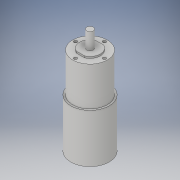
# Autodesk Inventor part: IG42-017
Saved by Autodesk Inventor 2019 (Build 230136000, 136)
## iProperties
Created: 2018-10-30
Part Number: IG42-017
Material: 一般
Document SubType Name: Modeling
Designer: kouki
Density: 1 g/cm^3
Appearance: 既定
Author: kouki
Autodesk Inventor part; units mm, degrees
ref_plane "YZ Plane" through (0, 0, 0) normal (1, 0, 0) x (0, 1, 0)
ref_plane "XZ Plane" through (0, 0, 0) normal (0, 1, 0) x (-1, 0, 0)
ref_plane "XY Plane" through (0, 0, 0) normal (0, 0, 1) x (1, 0, 0)
sketch "スケッチ1" plane through (0, 0, 0) normal (0, 1, 0) x (-1, 0, 0)
  circle A0 centre (0, 0) radius 21
  dimension "d0" = 42
  constraints: 1 centre point, 1 coincident
  measures "d0" diameter of A0
extrude "押し出し1" add sketch "スケッチ1" along normal blind 47
sketch "スケッチ2" plane through (0, 47, 0) normal (0, 1, 0) x (1, 0, 0)
  line L0 (0, 0) -> (0, 11.5)
  line L1 (0, 11.5) -> (0, -11.5)
  line L2 (-4.899, -11.5) -> (4.899, -11.5)
  line L3 (-4.899, 11.5) -> (4.899, 11.5)
  arc A0 (-4.899, 11.5) -> (-4.899, -11.5) centre (0, 0) ccw
  arc A1 (4.899, -11.5) -> (4.899, 11.5) centre (0, 0) ccw
  constraints: 8 end point, 4 point on circle, 2 centre point, 2 midpoint, 1 coincident, 1 horizontal, 1 perpendicular, 1 point on line, 1 vertical
extrude "押し出し2" add sketch "スケッチ2" along normal blind 2
sketch "スケッチ3" plane through (0, 47, 0) normal (0, 1, 0) x (1, 0, 0)
  circle A0 centre (0, 0) radius 17.5
  point P0 (-17.5, 0)
  point P1 (0, 17.5)
  point P2 (0, -17.5)
  point P3 (17.5, 0)
  dimension "d8" = 35
  constraints: 4 point on circle, 1 centre point, 1 coincident
  measures "d8" diameter of A0
hole "穴1" at (-17.5, 47, 0) at (0, 47, -17.5) at (0, 47, 17.5) at (17.5, 47, 0) direction (0, -1, 0) diameter 4 end through all
sketch "スケッチ4" plane through (0, 49, 0) normal (0, 1, 0) x (1, 0, 0)
  circle A0 centre (0, 0) radius 4
  dimension "d16" = 8
  constraints: 1 centre point, 1 coincident
  measures "d16" diameter of A0
extrude "押し出し3" add sketch "スケッチ4" along normal blind 20
sketch "スケッチ5" plane through (0, 0, 0) normal (0, -1, 0) x (1, 0, 0)
  circle A0 centre (0, 0) radius 23.25
  dimension "d19" = 46.5
  constraints: 1 centre point, 1 coincident
  measures "d19" diameter of A0
extrude "押し出し4" add sketch "スケッチ5" along normal blind 59
